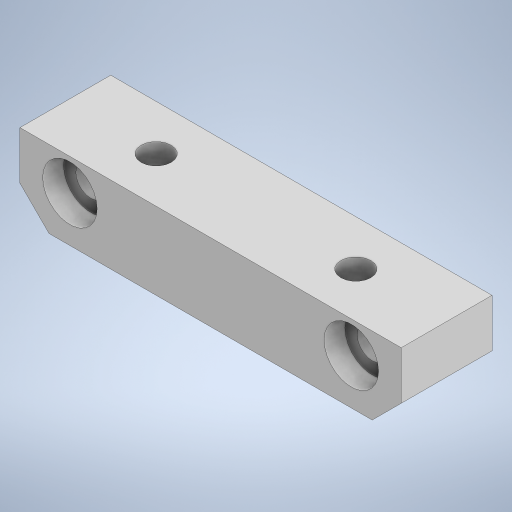
# Autodesk Inventor part: y_motor_lock_bottom2
Saved by Autodesk Inventor 2023 (Build 270158030, 158C)
## iProperties
Created: 2022-05-11
Part Number: y_motor_lock_bottom2
Material: 一般
Document SubType Name: Modeling
Designer: user
Density: 1 g/cm^3
Appearance: 預設
Author: user
## iProperties of the stored document y_motor_lock_bottom2_3D 列印.ipt
Created: 2022-05-15
Part Number: y_motor_lock_bottom2_3D 列印
Material: 一般
Document SubType Name: Modeling
Designer: user
Density: 1 g/cm^3
Appearance: 預設
Author: user
Autodesk Inventor part; units mm, degrees
ref_plane "YZ Plane" through (0, 0, 0) normal (1, 0, 0) x (0, 1, 0)
ref_plane "XZ Plane" through (0, 0, 0) normal (0, 1, 0) x (-1, 0, 0)
ref_plane "XY Plane" through (0, 0, 0) normal (0, 0, 1) x (1, 0, 0)
sketch "草圖1" plane through (0, 0, 0) normal (0, 0, 1) x (1, 0, 0)
  line L0 (-29.4, 0) -> (29.4, 0) projected
  line L1 (0, -5.95) -> (0, 5.95) projected
  line L2 (-21, 4.25) -> (21, 4.25)
  line L3 (21, 4.25) -> (21, -4.25)
  line L4 (21, -4.25) -> (-21, -4.25)
  line L5 (-21, -4.25) -> (-21, 4.25)
  point P0 (0, 0)
  dimension "d0" = 8.5
  dimension "d1" = 42
  constraints: 8 end point, 2 parallel, 1 horizontal, 1 perpendicular, 2 other
  measures "d0" distance of L4.end L2.start
  measures "d1" distance of L2.start L2.end
extrude "擠出1" add sketch "草圖1" along normal blind 10
sketch "草圖2" plane through (-21, -4.25, 0) normal (0, -1, 0) x (1, 0, 0)
  line L0 (0, 0) -> (42, 0) projected
  line L1 (42, 0) -> (42, 10) projected
  line L2 (0, 10) -> (42, 10) projected
  line L3 (0, 0) -> (0, 10) projected
  circle A0 centre (10, 5) radius 4
  circle A1 centre (10, 5) radius 1.65
  line L4 (21, 0) -> (21, -1.5889)
  circle A2 centre (32, 5) radius 4
  circle A3 centre (32, 5) radius 1.65
  line L5 (10, 1.7091) -> (7.15, 3.3546)
  line L6 (7.15, 3.3546) -> (7.15, 6.6454)
  line L7 (7.15, 6.6454) -> (10, 8.2909)
  line L8 (10, 8.2909) -> (12.85, 6.6454)
  line L9 (12.85, 6.6454) -> (12.85, 3.3546)
  line L10 (12.85, 3.3546) -> (10, 1.7091)
  line L11 (32, 1.7091) -> (29.15, 3.3546)
  line L12 (29.15, 3.3546) -> (29.15, 6.6454)
  line L13 (29.15, 6.6454) -> (32, 8.2909)
  line L14 (32, 8.2909) -> (34.85, 6.6454)
  line L15 (34.85, 6.6454) -> (34.85, 3.3546)
  line L16 (34.85, 3.3546) -> (32, 1.7091)
  point P0 (29.15, 5)
  dimension "d5" = 3.3
  dimension "d6" = 10
  dimension "d24" = 5.7
  dimension "d25" = 5.7
  dimension "d32" = 5
  constraints: 26 end point, 4 centre point, 3 coincident, 2 symmetric about line, 1 midpoint, 1 vertical, 28 other
  measures "d5" diameter of A1
  measures "d6" distance from line of L3 A0.centre
  measures "d24" distance between parallel lines of L9 L6
  measures "d25" distance from line of L15 point (29.15, 5)
  measures "d32" distance from line of L0 A0.centre
extrude "擠出2" cut sketch "草圖2" against normal blind 10 contours A1 | A3
sketch "草圖3" plane through (0, 0, 10) normal (0, 0, 1) x (1, 0, 0)
  line L0 (-21, -4.25) -> (21, -4.25) projected
  line L1 (21, -4.25) -> (21, 4.25) projected
  line L2 (21, 4.25) -> (-21, 4.25) projected
  line L3 (-21, 4.25) -> (-21, -4.25) projected
  line L4 (-17.8, -4.25) -> (-21, -1.05)
  line L5 (0, 4.25) -> (0, 6.2817)
  line L6 (17.8, -4.25) -> (21, -1.05)
  line L7 (17.8, -4.25) -> (22.3255, -4.25) construction
  circle A0 centre (-15.5, 0.75) radius 1.65
  circle A1 centre (-15.5, 0.75) radius 3
  circle A2 centre (15.5, 0.75) radius 1.65
  circle A3 centre (15.5, 0.75) radius 3
  line L8 (-18.5, 0.75) -> (-12.5, 0.75)
  line L9 (-12.5, 0.75) -> (-12.5, 4.25)
  line L10 (-12.5, 4.25) -> (-18.5, 4.25)
  line L11 (-18.5, 4.25) -> (-18.5, 0.75)
  line L12 (12.5, 0.75) -> (18.5, 0.75)
  line L13 (18.5, 0.75) -> (18.5, 4.25)
  line L14 (18.5, 4.25) -> (12.5, 4.25)
  line L15 (12.5, 4.25) -> (12.5, 0.75)
  point P0 (0, 0)
  point P1 (13.85, 0.75)
  point P2 (17.15, 0.75)
  point P3 (12.5, 4.25)
  point P4 (-12.5, 0.75)
  point P5 (-17.15, 0.75)
  point P6 (-13.85, 0.75)
  dimension "d16" = 6
  dimension "d11" = 3.2
  dimension "d12" = 45
  dimension "d13" = 45
  dimension "d14" = 3.2
  dimension "d15" = 3.3
  dimension "d17" = 5.5
  dimension "d28" = 3.5
  constraints: 24 end point, 7 point on line, 5 vertical, 4 parallel, 3 horizontal, 2 centre point, 2 coincident, 2 perpendicular, 2 symmetric about line, 1 equal length, 1 midpoint, 7 other
  measures "d11" distance from line of L3 L4.start
  measures "d12" angle of L0 L4
  measures "d13" angle of L7 L6
  measures "d14" distance of L0.end L6.start
  measures "d15" diameter of A0
  measures "d17" distance from line of L3 A0.centre
  measures "d28" distance from line of L2 A0.centre
extrude "擠出4" cut sketch "草圖3" against normal up to surface (10 mm away) contours L3 L4 L0 | L6 L1 L0 | L8 A0 | A0 L8 | L12 A2 | A2 L12
extrude "擠出6" cut sketch "草圖3" against normal blind 2.3 contours L8 A0 A1 | A1 L8 A0 | A0 L8 | L12 A2 A3 | A3 L12 A2 | L12 A2 picked at (-15.1043, 1.2463) picked at (16.003, 1.1372)
extrude "擠出7" cut sketch "草圖2" against normal blind 3 contours A1 | A3 | L5 L6 L7 L8 L9 L10 | L11 L12 L13 L14 L15 L16
